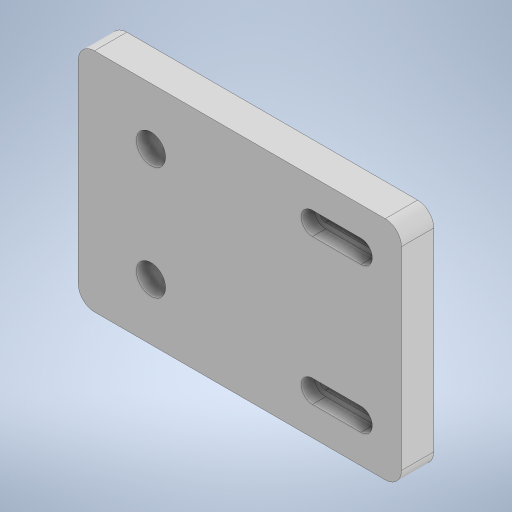
# Autodesk Inventor part: drzal_kamery_real_sense
Saved by Autodesk Inventor 2023 (Build 270158000, 158)
## iProperties
Created: 2025-01-13
Part Number: drzal_kamery_real_sense
Material: Všeobecné
Document SubType Name: Modeling
Designer: lisnik
Density: 1 g/cm^3
Appearance: Výchozí
Author: lisnik
Autodesk Inventor part; units mm, degrees
ref_plane "YZ Plane" through (0, 0, 0) normal (1, 0, 0) x (0, 1, 0)
ref_plane "XZ Plane" through (0, 0, 0) normal (0, 1, 0) x (-1, 0, 0)
ref_plane "XY Plane" through (0, 0, 0) normal (0, 0, 1) x (1, 0, 0)
sketch "Náčrt1" plane through (0, 0, 0) normal (0, 0, 1) x (1, 0, 0)
  line L0 (-70, 0) -> (70, 0) projected
  line L1 (0, -49) -> (0, 49) projected
  line L2 (-50, 35) -> (50, 35)
  line L3 (50, 35) -> (50, -35)
  line L4 (50, -35) -> (-50, -35)
  line L5 (-50, -35) -> (-50, 35)
  point P0 (0, 0)
  point P1 (0, 35)
  point P2 (-50, 0)
  dimension "d0" = 70
  dimension "d1" = 100
  constraints: 8 end point, 2 midpoint, 2 parallel, 2 point on line, 1 horizontal, 1 perpendicular
  measures "d0" distance between parallel lines of L4 L2
  measures "d1" distance between parallel lines of L3 L5
extrude "Vysunutí1" add sketch "Náčrt1" along normal blind 10
fillet "Zaoblení1" radius 5 4 edges at (50, 35, 5) (50, -35, 5) (-50, -35, 5) (-50, 35, 5)
sketch "Náčrt2" plane through (0, 0, 10) normal (0, 0, 1) x (1, 0, 0)
  line L0 (-50, 30) -> (-50, -30) projected
  point P0 (0, 0)
  point P1 (-27.5, 17.5)
  point P2 (-27.5, -17.5)
  point P3 (-50, 0)
  dimension "d5" = 22.5
  dimension "d6" = 22.5
  dimension "d7" = 35
  dimension "d8" = 17.5
  constraints: 1 midpoint
  measures "d5" distance from line of L0 point (-27.5, 17.5)
  measures "d6" distance from line of point (-27.5, -17.5) L0
  measures "d7" distance of point (-27.5, 17.5) point (-27.5, -17.5)
  measures "d8" vertical distance of point (-50, 0) point (-27.5, 17.5)
hole "Díra1" at (-27.5, 17.5, 10) at (-27.5, -17.5, 10) direction (0, 0, -1) diameter 9 end through all
sketch "Náčrt3" plane through (0, 0, 10) normal (0, 0, 1) x (1, 0, 0)
  line L0 (50, -30) -> (50, 30) projected
  line L1 (37.5, 22.5) -> (22.5, 22.5) construction
  line L2 (37.5, 26) -> (22.5, 26)
  line L3 (22.5, 19) -> (37.5, 19)
  arc A0 (37.5, 19) -> (37.5, 26) centre (37.5, 22.5) ccw
  arc A1 (22.5, 26) -> (22.5, 19) centre (22.5, 22.5) ccw
  line L4 (37.5, -22.5) -> (22.5, -22.5) construction
  line L5 (37.5, -19) -> (22.5, -19)
  line L6 (22.5, -26) -> (37.5, -26)
  arc A2 (37.5, -26) -> (37.5, -19) centre (37.5, -22.5) ccw
  arc A3 (22.5, -19) -> (22.5, -26) centre (22.5, -22.5) ccw
  point P0 (0, 0)
  point P1 (50, 0)
  point P2 (30, 22.5)
  point P3 (30, -22.5)
  dimension "d16" = 45
  dimension "d17" = 22.5
  dimension "d18" = 12.5
  dimension "d19" = 12.5
  dimension "d20" = 15
  dimension "d21" = 7
  dimension "d22" = 15
  dimension "d23" = 7
  constraints: 16 end point, 8 point on circle, 8 tangent, 4 centre point, 3 midpoint, 3 parallel, 1 perpendicular
  measures "d16" distance of L4.start L1.start
  measures "d17" vertical distance of point (50, 0) L4.start
  measures "d18" distance from line of L0 L4.start
  measures "d19" distance from line of L1.start L0
  measures "d20" distance of L1.start L1.end
  measures "d21" diameter of A1
  measures "d22" distance of L4.start L4.end
  measures "d23" diameter of A3
hole "Díra2" at (37.5, 22.5, 10) at (37.5, -22.5, 10) direction (0, 0, -1) diameter 3.4 end through all clearance for "Šroub se zápustnou hlavou ISO 2009/7046" size "M3" standard "ISO"
extrude "Vysunutí2" cut sketch "Náčrt3" against normal blind 4
sketch "Náčrt4" plane through (0, 0, 10) normal (0, 0, 1) x (1, 0, 0)
  circle A0 centre (37.5, 22.5) radius 1.7 projected
  arc A1 (22.5, 26) -> (22.5, 19) centre (22.5, 22.5) ccw projected
  line L0 (37.5, 22.5) -> (22.5, 22.5) construction
  line L1 (37.5, 20.8) -> (22.5, 20.8)
  line L2 (22.5, 24.2) -> (37.5, 24.2)
  arc A2 (37.5, 20.8) -> (37.5, 24.2) centre (37.5, 22.5) ccw
  arc A3 (22.5, 24.2) -> (22.5, 20.8) centre (22.5, 22.5) ccw
  circle A4 centre (37.5, -22.5) radius 1.7 projected
  line L3 (37.5, -22.5) -> (22.5, -22.5) construction
  line L4 (37.5, -24.2) -> (22.5, -24.2)
  line L5 (22.5, -20.8) -> (37.5, -20.8)
  arc A5 (37.5, -24.2) -> (37.5, -20.8) centre (37.5, -22.5) ccw
  arc A6 (22.5, -20.8) -> (22.5, -24.2) centre (22.5, -22.5) ccw
  arc A7 (22.5, -19) -> (22.5, -26) centre (22.5, -22.5) ccw projected
  point P0 (0, 0)
  point P1 (30, 22.5)
  point P2 (30, -22.5)
  constraints: 16 end point, 10 point on circle, 8 tangent, 4 centre point, 3 parallel, 2 midpoint, 1 coincident
extrude "Vysunutí3" cut sketch "Náčrt4" against normal through all
